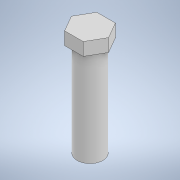
# Autodesk Inventor part: trail 13
Saved by Autodesk Inventor 2020.2 (Build 242310000, 310)
## iProperties
Created: 2020-02-27
Part Number: trail 13
Material: Generic
Document SubType Name: Modeling
Designer: lenovo
Density: 1 g/cm^3
Appearance: Default
Author: lenovo
Autodesk Inventor part; units mm, degrees
ref_plane "YZ Plane" through (0, 0, 0) normal (1, 0, 0) x (0, 1, 0)
ref_plane "XZ Plane" through (0, 0, 0) normal (0, 1, 0) x (-1, 0, 0)
ref_plane "XY Plane" through (0, 0, 0) normal (0, 0, 1) x (1, 0, 0)
sketch "Sketch1" plane through (0, 0, 0) normal (0, 1, 0) x (-1, 0, 0)
  circle A0 centre (0, 0) radius 2
  dimension "d0" = 4
  constraints: 1 centre point, 1 coincident
  measures "d0" diameter of A0
extrude "Extrusion1" add sketch "Sketch1" along normal blind 15
sketch "Sketch2" plane through (0, 15, 0) normal (0, 1, 0) x (1, 0, 0)
  line L0 (-1.4434, -2.5) -> (-2.8868, 0)
  line L1 (-2.8868, 0) -> (-1.4434, 2.5)
  line L2 (-1.4434, 2.5) -> (1.4434, 2.5)
  line L3 (1.4434, 2.5) -> (2.8868, 0)
  line L4 (2.8868, 0) -> (1.4434, -2.5)
  line L5 (1.4434, -2.5) -> (-1.4434, -2.5)
  point P0 (0, 0)
  point P1 (0, 0)
  dimension "d3" = 5
  constraints: 12 end point, 1 coincident, 13 other
  measures "d3" distance between parallel lines of L2 L5
extrude "Extrusion2" add sketch "Sketch2" along normal blind 2
body "Solid1"
